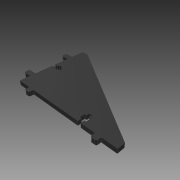
# Autodesk Inventor part: wiring_brace
Saved by Autodesk Inventor 2014 (Build 180170000, 170)
## iProperties
Created: 2013-12-07
Part Number: wiring_brace
Material: Generic
Document SubType Name: Modeling
Designer: buben
Density: 1 g/cm^3
Appearance: Anodized - Dark Gray
Author: buben
Subject: Laser Cutted
Autodesk Inventor part; units mm, degrees
ref_plane "YZ Plane" through (0, 0, 0) normal (1, 0, 0) x (0, 1, 0)
ref_plane "XZ Plane" through (0, 0, 0) normal (0, 1, 0) x (-1, 0, 0)
ref_plane "XY Plane" through (0, 0, 0) normal (0, 0, 1) x (1, 0, 0)
sketch "Sketch1" plane through (0, 0, 0) normal (0, 0, 1) x (1, 0, 0)
  line L0 (0, 106) -> (0, 0)
  line L1 (0, 0) -> (156.25, 0)
  line L2 (156.25, 0) -> (156.25, 10)
  line L3 (156.25, 10) -> (10, 106)
  line L4 (10, 106) -> (0, 106)
  dimension "d0" = 156.25
  dimension "d1" = 106
  dimension "d2" = 10
  dimension "d3" = 10
  constraints: 10 end point, 2 parallel, 1 perpendicular, 1 vertical
  measures "d0" distance of L0.end L1.end
  measures "d1" distance of L0.start L0.end
  measures "d2" distance of L3.end L0.start
  measures "d3" distance of L1.end L2.end
extrude "Extrusion1" add sketch "Sketch1" along normal blind 6.5
sketch "Sketch2" plane through (0, 0, 6.5) normal (0, 0, 1) x (1, 0, 0)
  line L0 (0, 106) -> (0, 0) projected
  line L1 (0, 0) -> (156.25, 0) projected
  line L2 (156.25, 0) -> (156.25, 10) projected
  line L3 (16.3, 55.25) -> (16.3, 50.75)
  line L4 (0, 50.75) -> (0, 55.25)
  line L5 (5, 57.75) -> (12.3, 57.75)
  line L6 (12.3, 48.25) -> (5, 48.25)
  line L7 (0, 55.25) -> (5, 55.25)
  line L8 (12.3, 55.25) -> (16.3, 55.25)
  line L9 (16.3, 50.75) -> (12.3, 50.75)
  line L10 (5, 50.75) -> (0, 50.75)
  line L11 (5, 48.25) -> (5, 50.75)
  line L12 (5, 55.25) -> (5, 57.75)
  line L13 (12.3, 57.75) -> (12.3, 55.25)
  line L14 (12.3, 50.75) -> (12.3, 48.25)
  line L15 (104, 16.3) -> (108.5, 16.3)
  line L16 (108.5, 0) -> (104, 0)
  line L17 (111, 12.3) -> (111, 5)
  line L18 (101.5, 5) -> (101.5, 12.3)
  line L19 (101.5, 12.3) -> (104, 12.3)
  line L20 (108.5, 12.3) -> (111, 12.3)
  line L21 (111, 5) -> (108.5, 5)
  line L22 (104, 5) -> (101.5, 5)
  line L23 (104, 0) -> (104, 5)
  line L24 (104, 12.3) -> (104, 16.3)
  line L25 (108.5, 16.3) -> (108.5, 12.3)
  line L26 (108.5, 5) -> (108.5, 0)
  point P0 (16.3, 53)
  point P1 (0, 53)
  point P2 (106.25, 16.3)
  dimension "d6" = 4.5
  dimension "d7" = 2.5
  dimension "d8" = 2.5
  dimension "d9" = 5
  dimension "d10" = 7.3
  dimension "d11" = 4
  dimension "d12" = 4.5
  dimension "d13" = 5
  dimension "d14" = 7.3
  dimension "d15" = 4
  dimension "d16" = 2.5
  dimension "d17" = 2.5
  dimension "d18" = 50
  constraints: 48 end point, 20 parallel, 10 collinear, 8 perpendicular, 6 horizontal, 3 midpoint, 1 horizontal alignment
  measures "d6" distance of L3.start L3.end
  measures "d7" distance of L5.end L8.start
  measures "d8" distance of L9.end L6.start
  measures "d9" distance of L10.start L4.start
  measures "d10" distance of L6.start L6.end
  measures "d11" distance of L3.end L9.end
  measures "d12" distance of L15.start L15.end
  measures "d13" distance of L16.end L22.start
  measures "d14" distance of L18.start L18.end
  measures "d15" distance of L19.end L15.start
  measures "d16" distance of L18.end L19.end
  measures "d17" distance of L20.start L17.start
  measures "d18" distance from line of L2 point (106.25, 16.3)
extrude "Extrusion2" cut sketch "Sketch2" against normal through all
sketch "Sketch3" plane through (0, 0, 6.5) normal (0, 0, 1) x (1, 0, 0)
  line L0 (0, 50.75) -> (0, 0) projected
  line L1 (0, 0) -> (104, 0) projected
  line L2 (108.5, 0) -> (156.25, 0) projected
  line L3 (10, 106) -> (0, 106) projected
  line L4 (0, 106) -> (0, 55.25) projected
  line L5 (0, 86) -> (-11, 86)
  line L6 (-13, 84) -> (-13, 80)
  line L7 (-11, 78) -> (0, 78)
  line L8 (0, 78) -> (0, 86)
  line L9 (0, 23) -> (-11, 23)
  line L10 (-13, 21) -> (-13, 17)
  line L11 (-11, 15) -> (0, 15)
  line L12 (0, 15) -> (0, 23)
  line L13 (20, 0) -> (28, 0)
  line L14 (28, 0) -> (28, -4.5)
  line L15 (26, -6.5) -> (22, -6.5)
  line L16 (20, -4.5) -> (20, 0)
  line L17 (128.25, 0) -> (136.25, 0)
  line L18 (136.25, 0) -> (136.25, -4.5)
  line L19 (134.25, -6.5) -> (130.25, -6.5)
  line L20 (128.25, -4.5) -> (128.25, 0)
  arc A0 (-11, 86) -> (-13, 84) centre (-11, 84) ccw
  arc A1 (-13, 80) -> (-11, 78) centre (-11, 80) ccw
  arc A2 (-11, 23) -> (-13, 21) centre (-11, 21) ccw
  arc A3 (-13, 17) -> (-11, 15) centre (-11, 17) ccw
  arc A4 (20, -4.5) -> (22, -6.5) centre (22, -4.5) ccw
  arc A5 (26, -6.5) -> (28, -4.5) centre (26, -4.5) ccw
  arc A6 (128.25, -4.5) -> (130.25, -6.5) centre (130.25, -4.5) ccw
  arc A7 (134.25, -6.5) -> (136.25, -4.5) centre (134.25, -4.5) ccw
  dimension "d21" = 2
  dimension "d22" = 8
  dimension "d23" = 8
  dimension "d24" = 8
  dimension "d25" = 8
  dimension "d26" = 13
  dimension "d27" = 6.5
  dimension "d28" = 15
  dimension "d29" = 20
  dimension "d30" = 20
  dimension "d31" = 20
  constraints: 32 end point, 16 point on circle, 16 tangent, 8 centre point, 8 parallel, 7 equal radius, 4 horizontal, 4 perpendicular, 4 point on line, 2 collinear
  measures "d21" radius of A0
  measures "d22" distance between parallel lines of L7 L5
  measures "d23" distance between parallel lines of L11 L9
  measures "d24" distance between parallel lines of L14 L16
  measures "d25" distance between parallel lines of L18 L20
  measures "d26" distance between parallel lines of L8 L6
  measures "d27" distance between parallel lines of L1 L15
  measures "d28" distance between parallel lines of L1 L11
  measures "d29" distance between parallel lines of L3 L5
  measures "d30" distance between parallel lines of L0 L16
  measures "d31" distance from line of L2.end L18
extrude "Extrusion3" add sketch "Sketch3" against normal blind 6.5
body "Solid1"
